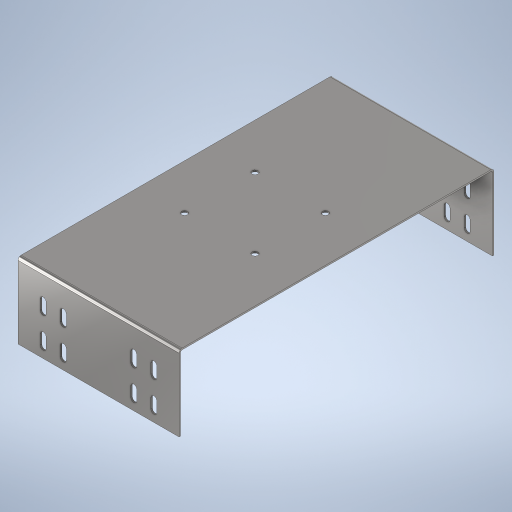
# Autodesk Inventor part: HCMUTE-CDT23-BAT_DO_BTC
Saved by Autodesk Inventor 2023 (Build 270158000, 158)
## iProperties
Created: 2023-10-30
Part Number: HCMUTE-CDT23-BAT_DO_BTC
Material: Stainless Steel
Document SubType Name: Sheet Metal
Designer: havie
Density: 8 g/cm^3
Sheet Metal Rule: Default_mm
Appearance: Semi-Polished
Mass: 1026.09 g
Surface Area: 1740.05 cm^2
Volume: 128.261 cm^3
Flat Pattern Width: 16 cm
Flat Pattern Length: 45.7786 cm
Flat Pattern Area: 732.457 cm^2
Sheet Metal Width: 160.000 mm
Sheet Metal Length: 457.786 mm
Sheet Metal Area: 73245.734 mm^2
Author: havie
Autodesk Inventor part; units mm, degrees
ref_plane "YZ Plane" through (0, 0, 0) normal (1, 0, 0) x (0, 1, 0)
ref_plane "XZ Plane" through (0, 0, 0) normal (0, 1, 0) x (-1, 0, 0)
ref_plane "XY Plane" through (0, 0, 0) normal (0, 0, 1) x (1, 0, 0)
sketch "Sketch4" plane through (0, 0, -0.75) normal (0, 0, -1) x (-1, 0, 0)
  circle A0 centre (-35, 49) radius 2.067 projected
  circle A1 centre (-35, 119) radius 2.067 projected
  circle A2 centre (35, 119) radius 2.067 projected
  circle A3 centre (35, 49) radius 2.067 projected
  circle A4 centre (-36, -51) radius 2.067 projected
  circle A5 centre (-36, -121) radius 2.067 projected
  circle A6 centre (34, -51) radius 2.067 projected
  circle A7 centre (34, -121) radius 2.067 projected
  point P0 (0, 0)
  constraints: 8 coincident
sketch "Sketch1" plane through (0, 0, 0) normal (0, 0, 1) x (1, 0, 0)
  line L0 (-95, 156.5) -> (95, 156.5)
  line L1 (95, 156.5) -> (95, -156.5)
  line L2 (95, -156.5) -> (-95, -156.5)
  line L3 (-95, -156.5) -> (-95, 156.5)
  line L4 (-95, 156.5) -> (95, -156.5) construction
  line L5 (95, 156.5) -> (-95, -156.5) construction
  point P0 (0, 0)
  dimension "d0" = 313
  dimension "d1" = 190
  measures "d0" distance of L2.end L0.start
  measures "d1" distance of L1.end L2.end
extrude "Plate1" add sketch "Sketch1" along normal mid plane 1.5
sketch "Sketch2" plane through (95, -155, -0.75) normal (0, -1, 0) x (1, 0, 0)
  line L0 (-190, 0) -> (0, 0)
  line L1 (0, 0) -> (0, 75)
  line L2 (0, 75) -> (-190, 75)
  line L3 (-190, 75) -> (-190, 0)
  constraints: 6 end point, 1 horizontal, 1 perpendicular, 1 vertical
edge flange "Flange1" height 75 angle 90 thickness 1.5 bend radius 1.5 thickness toward (0, -1, 0) relief straight relief width 1.5 relief depth 0.75 corner gap 1.5 corner form 0 edges at (0, -156.5, 0.75) (0, 156.5, 0.75) wall of the first edge with corners at (-95, -155, -0.75) (95, -155, -0.75) (95, -155, 74.25) (-95, -155, 74.25)
bend "Bend1"
corner "Corner1"
sketch "Sketch3" plane through (-95, -156.5, 74.25) normal (0, -1, 0) x (1, 0, 0)
  line L0 (40, -10) -> (40, -20) construction
  line L1 (37, -10) -> (37, -20)
  line L2 (43, -20) -> (43, -10)
  arc A0 (43, -10) -> (37, -10) centre (40, -10) ccw
  arc A1 (37, -20) -> (43, -20) centre (40, -20) ccw
  line L3 (0, 0) -> (190, 0) projected
  line L4 (0, -72) -> (0, 0) projected
  line L5 (60, -10) -> (60, -20) construction
  line L6 (57, -10) -> (57, -20)
  arc A2 (63, -10) -> (57, -10) centre (60, -10) ccw
  arc A3 (57, -20) -> (63, -20) centre (60, -20) ccw
  line L7 (63, -20) -> (63, -10)
  line L8 (40, -40) -> (40, -50) construction
  line L9 (37, -40) -> (37, -50)
  arc A4 (43, -40) -> (37, -40) centre (40, -40) ccw
  arc A5 (37, -50) -> (43, -50) centre (40, -50) ccw
  line L10 (43, -50) -> (43, -40)
  line L11 (60, -40) -> (60, -50) construction
  line L12 (57, -40) -> (57, -50)
  arc A6 (63, -40) -> (57, -40) centre (60, -40) ccw
  arc A7 (57, -50) -> (63, -50) centre (60, -50) ccw
  line L13 (63, -50) -> (63, -40)
  point P0 (95, -74.25)
  point P1 (40, -15)
  point P2 (37, -15)
  point P3 (57, -15)
  point P4 (60, -15)
  point P5 (37, -45)
  point P6 (40, -45)
  point P7 (57, -45)
  point P8 (60, -45)
  dimension "d13" = 10
  dimension "d14" = 6
  dimension "d15" = 15
  dimension "d16" = 40
  dimension "d19" = 20
  dimension "d22" = 30
  constraints: 32 end point, 16 point on circle, 8 centre point, 4 tangent, 2 midpoint, 2 vertical, 1 horizontal, 1 parallel, 39 other
  measures "d13" distance of L2.start L2.end
  measures "d14" distance from line of point (37, -15) L2
  measures "d15" distance from line of L3 point (40, -15)
  measures "d16" distance between parallel lines of L4 L0
  measures "d19" distance of L1.start L6.start
  measures "d22" distance of L1.start L9.start
extrude "Cut1" cut sketch "Sketch3" against normal through all
mirror "Mirror1" about plane through (0, 0, 0) normal (1, 0, 0) of "Cut1"
sketch "Sketch5" plane through (0, 0, -0.75) normal (0, 0, -1) x (-1, 0, 0)
  line L0 (222.4709, -155) -> (-377.5291, -155)
  point P0 (0, 0)
  point P1 (35, 36)
  point P2 (35, -34)
  point P3 (-35, -34)
  point P4 (-35, 36)
  dimension "d41" = 35
  dimension "d43" = 70
  dimension "d44" = 70
  dimension "d45" = 121
  constraints: 2 end point, 2 horizontal alignment, 2 vertical alignment, 1 horizontal, 2 other
  measures "d41" horizontal distance of point (35, 36) point (0, 0)
  measures "d43" distance of point (35, -34) point (35, 36)
  measures "d44" distance of point (-35, 36) point (35, 36)
  measures "d45" distance from line of L0 point (35, -34)
hole "Hole2" at (35, 36, -0.75) at (35, -34, -0.75) at (-35, -34, -0.75) at (-35, 36, -0.75) direction (0, 0, 1) diameter 6 end through all
sketch "Sketch6" plane through (-95, 156.5, 74.25) normal (0, 1, 0) x (1, 0, 0)
  line L0 (0, 0) -> (15, 0)
  line L1 (15, 0) -> (15, 100)
  line L2 (15, 100) -> (0, 100)
  line L3 (0, 100) -> (0, 0)
  line L4 (190, 0) -> (0, 0) projected
  line L5 (190, 0) -> (175, 0)
  line L6 (175, 0) -> (175, 100)
  line L7 (175, 100) -> (190, 100)
  line L8 (190, 100) -> (190, 0)
  point P0 (95, 74.25)
  dimension "d46" = 15
  dimension "d47" = 100
  dimension "d48" = 100
  dimension "d49" = 15
  constraints: 16 end point, 4 parallel, 2 horizontal, 2 perpendicular
  measures "d46" distance between parallel lines of L3 L1
  measures "d47" distance of L0.end L1.end
  measures "d48" distance of L5.end L6.end
  measures "d49" distance between parallel lines of L8 L6
extrude "Cut2" cut sketch "Sketch6" against normal blind 1000
equation "\"d25\" = Thickness"
equation "\"d39\" = Thickness"
equation "\"d2\" = Thickness"
equation "\"d3\" = BendReliefWidth"
equation "\"d4\" = BendReliefDepth"
equation "\"d5\" = MinimumRemnant"
equation "\"d6\" = TransitionRadius"
equation "\"d9\" = BendRadius"
equation "\"d10\" = CornerReliefSize"
equation "\"d11\" = GapSize"
equation "\"d12\" = JacobiRadiusSize"
equation "\"BendRadius\" = Thickness"
equation "\"BendReliefWidth\" = Thickness"
equation "\"BendReliefDepth\" = 0.5 * Thickness"
equation "\"CornerReliefSize\" = 4 * Thickness"
equation "\"MinimumRemnant\" = 2 * Thickness"
equation "\"TransitionRadius\" = BendRadius"
equation "\"JacobiRadiusSize\" = BendRadius"
equation "\"GapSize\" = Thickness"
equation "\"Thickness\" = 1.5"
body "Solid1"
